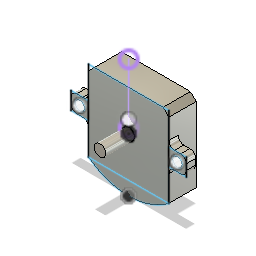
Micro Maus Motorhalterung (Autodesk Fusion 360 archive; units mm, degrees)
design "Motor"
Autodesk Fusion 360 part; units mm, degrees
note: some values were not read from the file. Chosen so that the rebuilt part matches the saved one: that a step has no effect.
sketch "Skizze1" plane through (0, 0, 0) normal (0, 0, 1) x (1, 0, 0)
  line L0 (-14, 14) -> (14, 14)
  line L1 (14, 14) -> (14, -14)
  line L2 (14, -14) -> (-14, -14)
  line L3 (-14, -14) -> (-14, 14)
  arc A0 (-14, -14) -> (14, -14) centre (0, 4.2566) ccw
  line L4 (-14, 3) -> (-20.1, 3)
  line L5 (-20.1, 3) -> (-20.1, -3)
  line L6 (-20.1, -3) -> (-14, -3)
  line L7 (-14, -3) -> (-14, 3)
  circle A1 centre (-17, 0) radius 1.6
  circle A2 centre (17, 0) radius 1.6
  line L8 (14, -3) -> (20.1, -3)
  line L9 (20.1, 3) -> (14, 3)
  line L10 (14, 3) -> (14, -3)
  line L11 (20.1, -3) -> (20.1, 3)
  line L12 (0, 1.75) -> (0, 22.5)
  circle A3 centre (0, 0) radius 2
  point P0 (0, -18.75)
  dimension "d16" = 40.2
  dimension "d17" = 28
  dimension "d18" = 6.1
  dimension "d21" = 4
  constraint horizontal L0
  constraint vertical L1
  constraint horizontal L2
  constraint vertical L3
  constraint coincident P0 A0
  constraint horizontal L4
  constraint vertical L5
  constraint horizontal L6
  constraint vertical L7
  constraint coincident L3 L4.start
  constraint horizontal L9
  constraint vertical L10
  constraint horizontal L8
  constraint vertical L11
  constraint collinear L1 L10
  constraint coincident A3.centre origin
  constraint symmetric L5 L11 L12
  measures "d16" distance of L5 L11
  measures "d17" distance of L1 L3
  measures "d18" distance of L10 L11
  measures "d21" diameter of A3
extrude "Extrusion1" add sketch "Skizze1" along normal blind 10 contours A3 makes body 1
extrude "Extrusion2" add sketch "Skizze1" against normal blind 9.5 separate body contours L0 L1 L2 L3 L7 L10 makes body 2
extrude "Extrusion3" add sketch "Skizze1" against normal blind 9.5 contours L2 A0 bodies 2
extrude "Extrusion4" add sketch "Skizze1" against normal blind 9.5 contours A3 bodies 1 2
extrude "Extrusion5" add sketch "Skizze1" against normal blind 3.2 contours L1 L8 L9 L10 L11 bodies 1
extrude "Extrusion6" add sketch "Skizze1" against normal blind 3.2 contours L3 L4 L5 L6 L7 bodies 1
chamfer "Fase1" distance 2 angle 45 1 edges at (14, 14, -4.75) on bodies 1
chamfer "Fase2" distance 2 angle 45 1 edges at (-14, 14, -4.75) on bodies 1
fillet "Abrundung1" radius 2 1 edges at (-14, 3, -1.6) on bodies 1
fillet "Abrundung2" radius 2 1 edges at (14, 3, -1.6) on bodies 1
fillet "Abrundung3" radius 2 1 edges at (14, -3, -1.6) on bodies 1
fillet "Abrundung4" radius 2 1 edges at (-14, -3, -1.6) on bodies 1
fillet "Abrundung5" radius 2 1 edges at (20.1, 3, -1.6) on bodies 1
fillet "Abrundung6" radius 2 1 edges at (20.1, -3, -1.6) on bodies 1
fillet "Abrundung7" radius 2 1 edges at (-20.1, 3, -1.6) on bodies 1
fillet "Abrundung8" radius 2 1 edges at (-20.1, -3, -1.6) on bodies 1

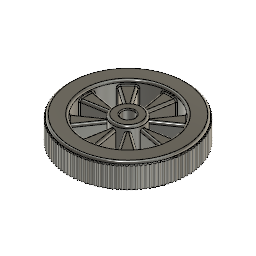
design "Reifen_Grip_V5"
part number: 2025-05-07-17-34-55-146
Autodesk Fusion 360 part; units mm, degrees
sketch "Skizze1" plane through (0, 0, 0) normal (0, 0, 1) x (1, 0, 0)
  circle A0 centre (0, 0) radius 19.5
  circle A1 centre (0, 0) radius 14
  circle A2 centre (0, 0) radius 5
  circle A3 centre (0, 0) radius 2.1
  line L0 (-13.8696, -1.9063) -> (-7.5114, -0.5773)
  line L1 (18.6418, -5.7214) -> (10.472, -4.0991)
  line L2 (10.472, -4.0991) -> (18.6418, -5.7214)
  line L3 (0.8682, 4.924) -> (2.4311, 13.7873)
  line L4 (-0.8682, 4.924) -> (-2.4311, 13.7873)
  line L5 (-3.3861, 19.2038) -> (-1.918, 10.8776)
  line L6 (-1.918, 10.8776) -> (-3.3861, 19.2038)
  line L7 (-2.4311, 13.7873) -> (-0.8682, 4.924)
  line L8 (-2.8679, 4.0958) -> (-8.0301, 11.4681)
  line L9 (-4.0958, 2.8679) -> (-11.4681, 8.0301)
  line L10 (-4.924, 0.8682) -> (-13.7873, 2.4311)
  line L11 (-4.924, -0.8682) -> (-13.7873, -2.4311)
  line L12 (4.924, -0.8682) -> (13.7873, -2.4311)
  line L13 (4.924, 0.8682) -> (13.7873, 2.4311)
  line L14 (-0.8682, -4.924) -> (-2.4311, -13.7873)
  line L15 (0.8682, -4.924) -> (2.4311, -13.7873)
  line L16 (-2.8679, -4.0958) -> (-8.0301, -11.4681)
  line L17 (-4.0958, -2.8679) -> (-11.4681, -8.0301)
  line L18 (2.8211, -4.1281) -> (7.8991, -11.5587)
  line L19 (4.0629, -2.9143) -> (11.3761, -8.16)
  line L20 (4.0958, 2.8679) -> (11.4681, 8.0301)
  line L21 (2.8679, 4.0958) -> (8.0301, 11.4681)
  dimension "d1" = 39
  dimension "d2" = 28
  dimension "d3" = 10
  dimension "d4" = 4.2
  constraint coincident A0.centre A1.centre
  constraint concentric A0 A2
  constraint concentric A2 A3
  constraint coincident A1 L0.start
  constraint coincident A0 L1.start
  constraint parallel L4 L6
  constraint coincident A2 L4.start
  constraint coincident A2 L3.start
  constraint coincident A1 L4.end
  constraint coincident A0 L5.start
  constraint collinear L4 L5
  constraint collinear L6 L7
  constraint coincident A1 L3.end
  constraint coincident A2 L8.start
  constraint coincident A2 L9.start
  constraint coincident A1 L8.end
  constraint coincident A1 L9.end
  constraint coincident A2 L10.start
  constraint coincident A2 L11.start
  constraint coincident A1 L10.end
  constraint coincident A1 L11.end
  constraint coincident A2 L12.start
  constraint coincident A2 L13.start
  constraint coincident A1 L12.end
  constraint coincident A1 L13.end
  constraint coincident A1 L14.end
  constraint coincident A2 L14.start
  constraint coincident A1 L15.end
  constraint coincident A2 L15.start
  constraint coincident A2 L16.start
  constraint coincident A2 L17.start
  constraint coincident A1 L17.end
  constraint coincident A1 L16.end
  constraint coincident A2 L18.start
  constraint coincident A2 L19.start
  constraint coincident A1 L18.end
  constraint coincident A1 L19.end
  constraint coincident A2 L20.start
  constraint coincident A2 L21.start
  constraint coincident A1 L21.end
  constraint coincident A1 L20.end
  measures "d1" diameter of A0
  measures "d2" diameter of A1
  measures "d3" diameter of A2
  measures "d4" diameter of A3
extrude "Extrusion3" add sketch "Skizze1" along normal blind 4 contours A2 makes body 1
extrude "Extrusion4" add sketch "Skizze1" along normal blind 2.5 contours A1 A2 L3 L4 L5 L6 L7 | A1 A2 L8 L9 | A1 A2 L18 L19 | A1 A2 L12 L13 | A1 A2 L20 L21 | A1 A2 L10 L11 | A1 A2 L14 L15 | A1 A2 L16 L17 bodies 1
extrude "Extrusion5" add sketch "Skizze1" along normal blind 4 contours A0 A1 L1 L2 L5 L6 | A0 A1 L1 L2 L5 L6 bodies 1
fillet "Abrundung1" radius 0.7 19 edges at (1.6497, 9.3557, 2.5) (-1.6497, 9.3557, 2.5) (-5.449, 7.7819, 2.5) (-7.7819, 5.449, 2.5) (-9.3557, 1.6497, 2.5) (-9.3557, -1.6497, 2.5) (-7.7819, -5.449, 2.5) (-5.449, -7.7819, 2.5) (-1.6497, -9.3557, 2.5) (1.6497, -9.3557, 2.5) (5.3601, -7.8434, 2.5) (7.7195, -5.5371, 2.5) (9.3557, -1.6497, 2.5) (9.3557, 1.6497, 2.5) (7.7819, 5.449, 2.5) (5.449, 7.7819, 2.5) (-4.6616, -1.8081, 4) (-13.0526, 5.0626, 4) (-18.1804, -7.0515, 4) on bodies 1
fillet "Abrundung2" radius 0.35 40 edges at (2.4311, 13.7873, 0.9) (2.2288, 13.8214, 2.2951) (0, 14, 2.5) (-2.2288, 13.8214, 2.2951) (-2.4311, 13.7873, 0.9) (-8.0301, 11.4681, 0.9) (-8.1972, 11.3492, 2.2951) (-9.8995, 9.8995, 2.5) (-11.3492, 8.1972, 2.2951) (-11.4681, 8.0301, 0.9) (11.4681, 8.0301, 0.9) (11.3492, 8.1972, 2.2951) (9.8995, 9.8995, 2.5) (8.1972, 11.3492, 2.2951) (8.0301, 11.4681, 0.9) (-13.7873, 2.4311, 0.9) (-13.8214, 2.2288, 2.2951) (-14, 0, 2.5) (-13.8214, -2.2288, 2.2951) (-13.7873, -2.4311, 0.9) (-11.4681, -8.0301, 0.9) (-11.3492, -8.1972, 2.2951) (-9.8995, -9.8995, 2.5) (-8.1972, -11.3492, 2.2951) (-8.0301, -11.4681, 0.9) (-2.4311, -13.7873, 0.9) (-2.2288, -13.8214, 2.2951) (0, -14, 2.5) (2.2288, -13.8214, 2.2951) (2.4311, -13.7873, 0.9) (13.7873, -2.4311, 0.9) (13.8214, -2.2288, 2.2951) (14, 0, 2.5) (13.8214, 2.2288, 2.2951) (13.7873, 2.4311, 0.9) (7.8991, -11.5587, 0.9) (8.0677, -11.4417, 2.2951) (9.7863, -10.0114, 2.5) (11.2553, -8.3258, 2.2951) (11.3761, -8.16, 0.9) on bodies 1
fillet "Abrundung3" radius 0.3 1 edges at (-1.9579, 0.7594, 4) on bodies 1
ref_plane "Arbeitsebene1" through (0, 0, 0.3) normal (0, 0, 1) x (1, 0, 0)
sketch "Skizze3" plane through (0, 0, 0.3) normal (0, 0, 1) x (1, 0, 0)
extrude "Extrusion8" add 1 faces at (-7.7001, -7.2908, 0) along direction (0, 0, -1) blind 4 on bodies 1 bodies 1
extrude "Extrusion9" [no effect]
extrude "Extrusion10" [no effect]
sketch "Skizze4" plane through (0, 0, 0) normal (0, 0, 1) x (1, 0, 0)
  circle A0 centre (-19.5, 0) radius 0.4
  dimension "d92" = 0.8
  measures "d92" diameter of A0
extrude "Extrusion11" add sketch "Skizze4" against normal blind 3.9 separate body makes body 2
extrude "Extrusion12" add 1 faces at (-19.4169, 0.2199, 0) along direction (0, 0, 1) blind 3 on bodies 2 bodies 2
pattern_circular "C-Anordnung2" count 110 over 360 about axis through (0, 0, -4) along (0, 0, 1) of bodies 2 makes body 3 at (-19.3627, -0.7274, -1.6) makes body 4 at (-19.2896, -1.8316, -1.6) makes body 5 at (-19.4725, -3.6308, -1.6) makes body 6 at (-19.1831, -4.7688, -1.6) makes body 7 at (-18.8132, -5.1073, -1.6) makes body 8 at (-18.6134, -6.2387, -1.6) makes body 9 at (-17.8349, -7.2115, -1.6) makes body 10 at (-17.8201, -8.3649, -1.6) makes body 11 at (-17.1675, -9.2357, -1.6) makes body 12 at (-16.3836, -10.143, -1.6) makes body 13 at (-15.9827, -11.8042, -1.6) makes body 14 at (-15.3085, -12.005, -1.6) makes body 15 at (-14.0586, -12.93, -1.6) makes body 16 at (-13.1923, -13.9435, -1.6) makes body 17 at (-12.4931, -14.4482, -1.6) makes body 18 at (-11.6479, -15.1379, -1.6) makes body 19 at (-11.3918, -16.2045, -1.6) makes body 20 at (-10.297, -16.3696, -1.6) makes body 21 at (-8.8959, -16.9024, -1.6) makes body 22 at (-7.7053, -17.7992, 0.7) makes body 23 at (-7.3548, -17.8858, -1.6) makes body 24 at (-5.7353, -18.2706, -1.6) makes body 25 at (-5.2681, -18.6076, -1.6) makes body 26 at (-4.2576, -19.2198, -1.6) makes body 27 at (-3.1386, -19.4685, -1.6) makes body 28 at (-1.2822, -19.5314, 0.7) makes body 29 at (-0.8748, -19.2494, -1.6) makes body 30 at (0.8642, -19.748, -1.6) makes body 31 at (1.9902, -19.6665, -1.6) makes body 32 at (2.4204, -19.1166, -1.6) makes body 33 at (4.098, -19.442, -1.6) makes body 34 at (4.6594, -19.1263, -1.6) makes body 35 at (6.4207, -18.6092, 0.7) makes body 36 at (7.3548, -17.8858, 0.7) makes body 37 at (7.7028, -17.7795, -1.6) makes body 38 at (8.9312, -16.8838, -1.6) makes body 39 at (9.8592, -17.0389, -1.6) makes body 40 at (11.3915, -15.9878, 0.7) makes body 41 at (11.6795, -15.1136, -1.6) makes body 42 at (12.6203, -15.1081, -1.6) makes body 43 at (13.9882, -14.0246, -1.6) makes body 44 at (14.0856, -12.9006, -1.6) makes body 45 at (14.7991, -12.0754, -1.6) makes body 46 at (15.9294, -11.8312, -1.6) makes body 47 at (16.4054, -10.9425, -1.6) makes body 48 at (17.3575, -9.4578, -1.6) makes body 49 at (17.1908, -8.8584, -1.6) makes body 50 at (17.6017, -7.4169, -1.6) makes body 51 at (18.1186, -6.8673, -1.6) makes body 52 at (18.5879, -5.8747, -1.6) makes body 53 at (19.1285, -4.7931, -1.6) makes body 54 at (18.9563, -3.0196, -1.6) makes body 55 at (19.4562, -2.6141, -1.6) makes body 56 at (19.797, -1.341, -1.6) makes body 57 at (19.49, -0.3999, -1.6) makes body 58 at (19.3627, 0.7274, -1.6) makes body 59 at (19.2896, 1.8316, -1.6) makes body 60 at (19.4725, 3.6308, -1.6) makes body 61 at (19.1831, 4.7688, -1.6) makes body 62 at (18.8132, 5.1073, -1.6) makes body 63 at (18.5462, 6.1959, -1.6) makes body 64 at (18.2409, 7.8774, -1.6) makes body 65 at (17.8201, 8.3649, -1.6) makes body 66 at (17.1675, 9.2357, -1.6) makes body 67 at (16.0576, 10.3433, -1.6) makes body 68 at (15.4409, 11.2431, -1.6) makes body 69 at (15.3085, 12.005, -1.6) makes body 70 at (14.0586, 12.93, -1.6) makes body 71 at (13.9727, 13.8669, -1.6) makes body 72 at (12.9376, 14.374, -1.6) makes body 73 at (12.0662, 15.8093, -1.6) makes body 74 at (11.3918, 16.2045, -1.6) makes body 75 at (9.7585, 16.4476, -1.6) makes body 76 at (8.8959, 16.9024, -1.6) makes body 77 at (7.7053, 17.7992, 0.7) makes body 78 at (7.3548, 17.8858, -1.6) makes body 79 at (5.7353, 18.2706, -1.6) makes body 80 at (4.6875, 19.1547, -1.6) makes body 81 at (3.5599, 19.3611, 0.7) makes body 82 at (3.1386, 19.4685, -1.6) makes body 83 at (1.2822, 19.5314, 0.7) makes body 84 at (0.8748, 19.2494, -1.6) makes body 85 at (-0.8642, 19.748, -1.6) makes body 86 at (-1.9902, 19.6665, -1.6) makes body 87 at (-2.4204, 19.1166, -1.6) makes body 88 at (-3.647, 18.7812, -1.6) makes body 89 at (-4.6594, 19.1263, -1.6) makes body 90 at (-6.3163, 18.8206, -1.6) makes body 91 at (-7.3548, 17.8858, 0.7) makes body 92 at (-7.7028, 17.7795, -1.6) makes body 93 at (-8.7296, 17.0954, -1.6) makes body 94 at (-9.8592, 17.0389, -1.6) makes body 95 at (-10.6214, 15.9889, -1.6) makes body 96 at (-11.6795, 15.1136, -1.6) makes body 97 at (-12.6203, 15.1081, -1.6) makes body 98 at (-13.3262, 13.6837, -1.6) makes body 99 at (-14.0856, 12.9006, -1.6) makes body 100 at (-14.883, 12.6825, -1.6) makes body 101 at (-15.9294, 11.8312, -1.6) makes body 102 at (-16.4054, 10.9425, -1.6) makes body 103 at (-17.3575, 9.4578, -1.6) makes body 104 at (-17.1908, 8.8584, -1.6) makes body 105 at (-18.1077, 7.9632, -1.6) makes body 106 at (-18.1186, 6.8673, -1.6) makes body 107 at (-18.9788, 5.7901, -1.6) makes body 108 at (-19.1285, 4.7931, -1.6) makes body 109 at (-18.9563, 3.0196, -1.6) makes body 110 at (-19.3687, 1.8229, 0.7) makes body 111 at (-19.797, 1.341, -1.6)
extrude "Extrusion6" [suppressed]
fillet "Abrundung4" [suppressed]
pattern_circular "C-Anordnung1" [suppressed]
extrude "Extrusion7" [suppressed]
